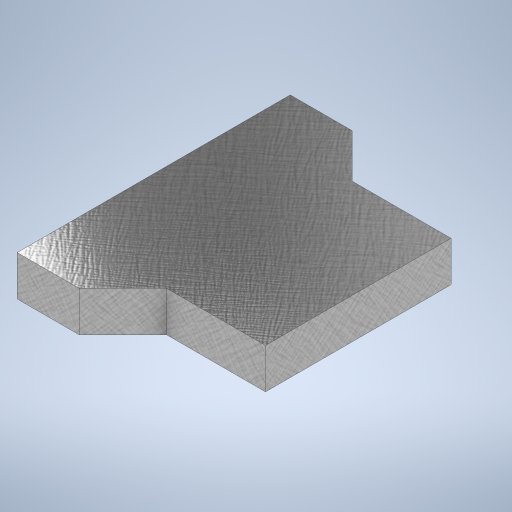
# Autodesk Inventor part: union_movllantas
Saved by Autodesk Inventor 2024 (Build 280153000, 153)
## iProperties
Created: 2023-05-07
Part Number: union_movllantas
Material: Generic
Document SubType Name: Modeling
Designer: Diego
Density: 1 g/cm^3
Appearance: Default
Author: Diego
Autodesk Inventor part; units mm, degrees
ref_plane "YZ Plane" through (0, 0, 0) normal (1, 0, 0) x (0, 1, 0)
ref_plane "XZ Plane" through (0, 0, 0) normal (0, 1, 0) x (-1, 0, 0)
ref_plane "XY Plane" through (0, 0, 0) normal (0, 0, 1) x (1, 0, 0)
sketch "Sketch1" plane through (0, 0, 0) normal (0, 1, 0) x (-1, 0, 0)
  point P0 (0, 0)
sketch "Sketch2" plane through (0, 0, 0) normal (0, 1, 0) x (-1, 0, 0)
  line L0 (0, 0) -> (0, 15)
  line L1 (0, 15) -> (8, 15)
  line L2 (8, 15) -> (11.5355, 18.5355)
  line L3 (8, 15) -> (13, 15) construction
  line L4 (11.5355, 18.5355) -> (16.5355, 18.5355)
  line L5 (0, 7.5) -> (15.5, 7.5) construction
  line L6 (0, 0) -> (8, 0)
  line L7 (8, 0) -> (11.5355, -3.5355)
  line L8 (8, 0) -> (13, 0) construction
  line L9 (11.5355, -3.5355) -> (16.5355, -3.5355)
  line L10 (16.5355, 18.5355) -> (16.5355, -3.5355)
  dimension "d2" = 15
  dimension "d3" = 8
  dimension "d4" = 5
  dimension "d5" = 45
  dimension "d6" = 5
  constraints: 22 end point, 4 horizontal, 4 symmetric about line, 2 vertical, 1 equal length, 1 midpoint
  measures "d2" distance of L0.start L0.end
  measures "d3" distance of L0.end L1.end
  measures "d4" distance of L1.end L2.end
  measures "d5" angle of L3 L2
  measures "d6" distance of L2.end L4.end
extrude "Extrusion1" add sketch "Sketch2" along normal blind 3.25
body "Solid1"
